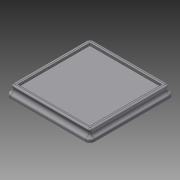
# Autodesk Inventor part: Board Piece 2
Saved by Autodesk Inventor 2015 SP1 (Build 190203100, 203)
## iProperties
Created: 2015-06-11
Part Number: Board Piece 2
Material: Generic
Document SubType Name: Modeling
Designer: Nathan
Density: 1 g/cm^3
Appearance: Default
Author: Nathan
Autodesk Inventor part; units mm, degrees
ref_plane "YZ Plane" through (0, 0, 0) normal (1, 0, 0) x (0, 1, 0)
ref_plane "XZ Plane" through (0, 0, 0) normal (0, 1, 0) x (-1, 0, 0)
ref_plane "XY Plane" through (0, 0, 0) normal (0, 0, 1) x (1, 0, 0)
sketch "Sketch2" plane through (0, 0, 0) normal (0, 1, 0) x (-1, 0, 0)
  line L0 (0.2, 188.9265) -> (379.8, 188.9265)
  line L1 (380, 188.7265) -> (380, -190.8735)
  line L2 (379.8, -191.0735) -> (0.2, -191.0735)
  line L3 (0, -190.8735) -> (0, 188.7265)
  arc A0 (0.2, 188.9265) -> (0, 188.7265) centre (0.2, 188.7265) ccw
  arc A1 (0, -190.8735) -> (0.2, -191.0735) centre (0.2, -190.8735) ccw
  arc A2 (379.8, -191.0735) -> (380, -190.8735) centre (379.8, -190.8735) ccw
  arc A3 (380, 188.7265) -> (379.8, 188.9265) centre (379.8, 188.7265) ccw
  point P0 (0, 0)
  point P1 (380, -191.0735)
  point P2 (380, 188.9265)
  point P3 (0, -191.0735)
  dimension "d1" = 380
  dimension "d2" = 380
  dimension "d3" = 0.2
  constraints: 8 end point, 8 point on circle, 8 tangent, 6 point on line, 4 centre point, 3 equal radius, 2 parallel, 1 horizontal, 1 perpendicular
  measures "d1" distance of point (380, -191.073) point (0, -191.073)
  measures "d2" distance of point (380, 188.927) point (380, -191.073)
  measures "d3" radius of A0
sketch "Sketch1" plane through (0, 0, 0) normal (0, 0, 1) x (1, 0, 0)
  line L0 (0, 0) -> (0, 50)
  line L1 (0, 50) -> (4.0204, 50) construction
  line L2 (4.0204, 50) -> (9.5242, 47.979) construction
  line L3 (9.5242, 47.979) -> (11.3737, 47.979) construction
  line L4 (11.3737, 47.979) -> (8.9562, 37.1523) construction
  line L5 (8.9562, 37.1523) -> (6.6334, 32.9423) construction
  line L6 (6.6334, 32.9423) -> (6.6334, 25) construction
  line L7 (6.6334, 25) -> (13.82, 14.5057) construction
  line L8 (13.82, 14.5057) -> (22.7474, 14.5057) construction
  line L9 (22.7474, 14.5057) -> (22.7474, 9.2795) construction
  line L10 (22.7474, 9.2795) -> (22.7474, 0) construction
  spline S0 degree 4 poles (0, 50) (4.0204, 50) (9.5242, 47.979) (11.3737, 47.979) (8.9562, 37.1523) (6.6334, 32.9423) (6.6334, 25) (13.82, 14.5057) (22.7474, 14.5057) (22.7474, 9.2795) (22.7474, 0) knots 1 1 1 1 1 2 3 4 5 6 7 8 8 8 8 8
  line L11 (0, 0) -> (22.7474, 0)
  dimension "d0" = 50
  constraints: 4 end point, 4 vertical, 1 horizontal, 1 perpendicular, 3 other
  measures "d0" distance of L0.start L0.end
sweep "Sweep1" add profiles "Sketch1" path "Sketch2"
extrude "Extrusion1" add sketch "Sketch2" along normal blind 50
sketch "Sketch3" plane through (0, 50, 0) normal (0, 1, 0) x (1, 0, 0)
  line L0 (-370, -180) -> (-10, -180)
  line L1 (-10, -180) -> (-10, 180)
  line L2 (-10, 180) -> (-370, 180)
  line L3 (-370, 180) -> (-370, -180)
  line L4 (-370, -180) -> (-10, 180) construction
  line L5 (-10, -180) -> (-370, 180) construction
  point P0 (0, 0)
  point P1 (-190, 0)
  dimension "d8" = 360
  dimension "d9" = 360
  constraints: 12 end point, 2 midpoint, 2 parallel, 1 horizontal, 1 perpendicular
  measures "d8" distance of L2.end L1.end
  measures "d9" distance of L1.end L0.end
extrude "Extrusion2" cut sketch "Sketch3" against normal blind 10
sketch "Sketch4" plane through (0, 50, 0) normal (0, 1, 0) x (1, 0, 0)
  line L0 (-370, -180) -> (-370, 180) projected
  line L1 (-370, 0) -> (-10, 0)
  line L2 (-10, 180) -> (-10, -180) projected
  line L3 (-372.5, -182.5) -> (-7.5, -182.5)
  line L4 (-7.5, -182.5) -> (-7.5, 182.5)
  line L5 (-7.5, 182.5) -> (-372.5, 182.5)
  line L6 (-372.5, 182.5) -> (-372.5, -182.5)
  line L7 (-372.5, -182.5) -> (-7.5, 182.5) construction
  line L8 (-7.5, -182.5) -> (-372.5, 182.5) construction
  point P0 (0, 0)
  point P1 (-190, 0)
  dimension "d12" = 365
  dimension "d13" = 365
  constraints: 14 end point, 5 midpoint, 2 parallel, 1 horizontal, 1 perpendicular
  measures "d12" distance of L5.end L4.end
  measures "d13" distance of L4.end L3.end
extrude "Extrusion3" cut sketch "Sketch4" against normal blind 2.5
body "Solid1"
